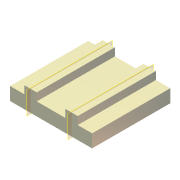
# Autodesk Inventor part: Lift Spacer
Saved by Autodesk Inventor 2011 (Build 150239000, 239)
## iProperties
Created: 2014-09-14
Part Number: Lift Spacer
Document SubType Name: Modeling
Designer: Family Room
Density: 1 g/cm^3
Author: Family Room
Autodesk Inventor part; units mm, degrees
ref_plane "YZ Plane" through (0, 0, 0) normal (1, 0, 0) x (0, 1, 0)
ref_plane "XZ Plane" through (0, 0, 0) normal (0, 1, 0) x (-1, 0, 0)
ref_plane "XY Plane" through (0, 0, 0) normal (0, 0, 1) x (1, 0, 0)
sketch "Sketch1" plane through (0, 0, 0) normal (0, 0, 1) x (1, 0, 0)
  line L0 (-24.1875, -2.5136) -> (15.8125, -2.5136)
  line L1 (15.8125, -2.5136) -> (15.8125, 3.8364)
  line L2 (-24.1875, 3.8364) -> (-24.1875, -2.5136)
  line L3 (-11.1875, 3.8364) -> (-11.1875, 7.6464)
  line L4 (-11.1875, 7.6464) -> (-17.1875, 7.6464)
  line L5 (-17.1875, 7.6464) -> (-17.1875, 3.8364)
  line L6 (-17.1875, 3.8364) -> (-24.1875, 3.8364)
  line L7 (8.8125, 3.8364) -> (8.8125, 7.6464)
  line L8 (8.8125, 7.6464) -> (2.8125, 7.6464)
  line L9 (2.8125, 7.6464) -> (2.8125, 3.8364)
  line L10 (15.8125, 3.8364) -> (8.8125, 3.8364)
  line L11 (2.8125, 3.8364) -> (-11.1875, 3.8364)
  point P0 (0, 0)
  dimension "d0" = 40
  dimension "d1" = 6.35
  dimension "d2" = 6
  dimension "d3" = 3.81
  dimension "d4" = 7
  dimension "d5" = 6
  dimension "d6" = 3.81
  dimension "d7" = 7
  constraints: 24 end point, 6 parallel, 1 horizontal, 1 perpendicular
  measures "d0" distance of L2.start L1.end
  measures "d1" distance of L1.end L0.end
  measures "d2" distance of L4.end L3.end
  measures "d3" distance of L3.end L3.start
  measures "d4" distance between parallel lines of L2 L5
  measures "d5" distance of L8.end L7.end
  measures "d6" distance of L7.end L7.start
  measures "d7" distance between parallel lines of L1 L7
extrude "Extrusion1" add sketch "Sketch1" along normal blind 38.1
ref_plane "Work Plane1" through (5.8125, 3.8364, 0) normal (1, 0, 0) x (0, 0, -1)
ref_plane "Work Plane2" through (-14.1875, 3.8364, 0) normal (1, 0, 0) x (0, 0, -1)
body "Solid1"
